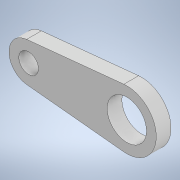
# Autodesk Inventor part: 1.5
Saved by Autodesk Inventor 2022 (Build 260153000, 153)
## iProperties
Created: 2023-04-17
Part Number: 1.5
Material: Genérico
Document SubType Name: Modeling
Designer: jpjoa
Density: 1 g/cm^3
Appearance: Padrão
Author: jpjoa
Autodesk Inventor part; units mm, degrees
ref_plane "YZ Plane" through (0, 0, 0) normal (1, 0, 0) x (0, 1, 0)
ref_plane "XZ Plane" through (0, 0, 0) normal (0, 1, 0) x (-1, 0, 0)
ref_plane "XY Plane" through (0, 0, 0) normal (0, 0, 1) x (1, 0, 0)
sketch "Esboço1" plane through (0, 0, 0) normal (0, 0, 1) x (1, 0, 0)
  circle A0 centre (0, 0) radius 10
  circle A1 centre (100, 0) radius 20
  circle A2 centre (0, 0) radius 20
  circle A3 centre (100, 0) radius 30
  line L0 (-2, -19.8997) -> (97, -29.8496)
  line L1 (-2, 19.8997) -> (97, 29.8496)
  dimension "d0" = 20
  dimension "d1" = 40
  dimension "d2" = 40
  dimension "d3" = 60
  dimension "d4" = 100
  dimension "d5" = 0
  dimension "d6" = 0
  constraints: 4 centre point, 4 end point, 4 point on circle, 4 tangent, 2 coincident, 1 horizontal alignment
  measures "d0" diameter of A0
  measures "d1" diameter of A1
  measures "d2" diameter of A2
  measures "d3" diameter of A3
  measures "d4" distance of A1.centre A0.centre
  measures "d5" distance of A0.centre point (0, 0)
  measures "d6" distance of point (0, 0) A0.centre
extrude "Extrusão1" add sketch "Esboço1" along normal blind 15
